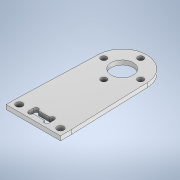
# Autodesk Inventor part: Foot_roll_vertical_02
Saved by Autodesk Inventor 2020 (Build 240168000, 168)
## iProperties
Created: 2021-09-15
Part Number: Foot_roll_vertical_02
Material: アルミニウム 2014-T4
Document SubType Name: Modeling
Designer: naoki
Density: 2.8 g/cm^3
Appearance: サテン
Author: naoki
Autodesk Inventor part; units mm, degrees
ref_plane "YZ Plane" through (0, 0, 0) normal (1, 0, 0) x (0, 1, 0)
ref_plane "XZ Plane" through (0, 0, 0) normal (0, 1, 0) x (-1, 0, 0)
ref_plane "XY Plane" through (0, 0, 0) normal (0, 0, 1) x (1, 0, 0)
sketch "スケッチ1" plane through (0, 0, 0) normal (0, 0, 1) x (1, 0, 0)
  line L0 (-63.6765, 0) -> (66.53, 0) construction
  line L1 (0, 73.5962) -> (0, -63.7716) construction
  circle A0 centre (0, 0) radius 5.05
  circle A1 centre (0, 0) radius 8 construction
  circle A2 centre (0, 0) radius 11.25
  circle A3 centre (0, 8.5) radius 1.35
  circle A4 centre (0, 8.5) radius 2.75 construction
  circle A5 centre (-8.5, 0) radius 2.75 construction
  circle A6 centre (-8.5, 0) radius 1.35
  circle A7 centre (0, -8.5) radius 2.75 construction
  circle A8 centre (0, -8.5) radius 1.35
  circle A9 centre (8.5, 0) radius 2.75 construction
  circle A10 centre (8.5, 0) radius 1.35
  line L2 (12.5, -41) -> (-12.5, -41)
  line L3 (-12.5, -41) -> (-12.5, -36)
  line L4 (-12.5, -36) -> (12.5, -36) construction
  line L5 (12.5, -36) -> (12.5, -41)
  line L6 (12.5, -41) -> (-12.5, -36) construction
  line L7 (-12.5, -41) -> (12.5, -36) construction
  line L8 (12.5, -36) -> (11.2433, 0.3883)
  line L9 (-12.5, -36) -> (-11.2433, 0.3883)
  circle A11 centre (-9.5, -38) radius 1.55
  line L10 (-12.5, -38) -> (12.5, -38) construction
  line L11 (-4.75, -36) -> (-4.75, -41) construction
  line L12 (4.75, -36) -> (4.75, -41) construction
  circle A12 centre (9.5, -38) radius 1.55
  line L13 (-4.75, -36) -> (4.75, -36) construction
  line L14 (4.75, -36) -> (4.75, -38.5) construction
  line L15 (4.75, -38.5) -> (-4.75, -38.5) construction
  line L16 (-4.75, -38.5) -> (-4.75, -36) construction
  line L17 (-4.75, -37.25) -> (4.75, -37.25) construction
  line L18 (-4.76, -38.51) -> (4.76, -38.51)
  line L19 (4.76, -38.51) -> (4.76, -35.99)
  line L20 (4.76, -35.99) -> (-4.76, -35.99)
  line L21 (-4.76, -35.99) -> (-4.76, -38.51)
  circle A13 centre (-3.71, -35.99) radius 1.05
  circle A14 centre (-3.71, -38.51) radius 1.05
  circle A15 centre (3.71, -35.99) radius 1.05
  circle A16 centre (3.71, -38.51) radius 1.05
  point P0 (0, -38.5)
  point P1 (4.75, -36)
  point P2 (2.66, -38.51)
  point P3 (-2.66, -38.51)
  point P4 (-2.66, -35.99)
  point P5 (2.66, -35.99)
  dimension "d0" = 10.1
  dimension "d1" = 16
  dimension "d4" = 2.7
  dimension "d5" = 8.5
  dimension "d6" = 5.5
  dimension "d7" = 22.5
  dimension "d10" = 360
  dimension "d12" = 25
  dimension "d13" = 5
  dimension "d14" = 36
  dimension "d15" = 3
  dimension "d16" = 9.5
  dimension "d17" = 3.1
  dimension "d18" = 3
  dimension "d19" = 4.75
  dimension "d30" = 19
  dimension "d39" = 0.01
  dimension "d40" = 1.05
  dimension "d41" = 2.1
  constraints: 44 end point, 17 centre point, 10 point on line, 9 coincident, 6 parallel, 5 midpoint, 5 perpendicular, 5 symmetric about line, 4 horizontal, 2 point on circle, 2 tangent, 1 vertical, 25 other
  measures "d0" diameter of A0
  measures "d1" diameter of A1
  measures "d4" diameter of A3
  measures "d5" distance from line of L0 A3.centre
  measures "d6" diameter of A4
  measures "d7" diameter of A2
  measures "d12" distance of L3.end L4.end
  measures "d13" distance of L2.end L3.end
  measures "d14" distance from line of point (0, 0) L4
  measures "d15" distance from line of L3 point (-9.5, -38)
  measures "d16" distance from line of L1 point (-9.5, -38)
  measures "d17" diameter of A11
  measures "d18" distance between parallel lines of L2 L10
  measures "d19" distance from line of L11 A11.centre
  measures "d30" distance of A11.centre A12.centre
  measures "d39" distance between parallel lines of L15 L18
  measures "d40" distance from line of L21 point (-3.71, -35.99)
  measures "d41" diameter of A13
extrude "押し出し1" add sketch "スケッチ1" along normal blind 2
equation "\"d19\" = 0.5 * d16"
